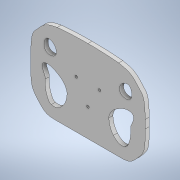
# Autodesk Inventor part: CF_base_3
Saved by Autodesk Inventor 2021 (Build 250183000, 183)
## iProperties
Created: 2020-12-19
Part Number: CF_base_3
Material: Generic
Document SubType Name: Modeling
Designer: capta
Density: 1 g/cm^3
Appearance: Default
Author: capta
Autodesk Inventor part; units mm, degrees
ref_plane "YZ Plane" through (0, 0, 0) normal (1, 0, 0) x (0, 1, 0)
ref_plane "XZ Plane" through (0, 0, 0) normal (0, 1, 0) x (-1, 0, 0)
ref_plane "XY Plane" through (0, 0, 0) normal (0, 0, 1) x (1, 0, 0)
sketch "Sketch1" plane through (0, 0, 0) normal (0, 0, 1) x (1, 0, 0)
  spline S0 degree 4 poles (-107.95, -1.5875) (-107.9501, -31.5854) (-105.1191, -42.7753) (-94.6432, -54.7155) (-85.2117, -65.4653) (-79.1753, -69.1153) (-72.5093, -71.2291) (-62.4463, -71.4375) knots 1 1 1 1 1 2 3 4 5 5 5 5 5
  line L0 (-62.4463, -71.4375) -> (62.4463, -71.4375)
  spline S1 degree 4 poles (62.4463, -71.4375) (72.5094, -71.2291) (79.1753, -69.1152) (85.2117, -65.4653) (94.6431, -54.7154) (105.119, -42.7752) (107.95, -31.5853) (107.95, -1.5875) knots 1 1 1 1 1 2 3 4 5 5 5 5 5
  spline S2 degree 4 poles (107.95, 14.2875) (107.3863, 39.342) (103.6451, 53.7014) (98.0708, 55.8562) (88.8552, 69.2477) (79.1753, 76.065) (71.1856, 78.9229) (57.9142, 81.444) knots 1 1 1 1 1 2 3 4 5 5 5 5 5
  spline S3 degree 2 poles (57.9142, 81.444) (34.5422, 83.9709) (0, 84.1375) knots 0 0 0 1 1 1
  spline S4 degree 2 poles (0, 84.1375) (-34.5422, 83.9709) (-57.9142, 81.444) knots 0 0 0 1 1 1
  spline S5 degree 4 poles (-57.9142, 81.444) (-71.1856, 78.9229) (-79.1753, 76.065) (-88.8553, 69.2477) (-98.0708, 55.8562) (-103.6451, 53.7014) (-107.3863, 39.342) (-107.95, 14.2875) knots 1 1 1 1 1 2 3 4 5 5 5 5 5
  circle A0 centre (21.971, 12.685) radius 2.3495
  circle A1 centre (0, -25.3699) radius 2.3495
  circle A2 centre (-21.971, 12.685) radius 2.3495
  spline S6 degree 3 poles (-80.6784, -14.2875) (-80.6812, -14.2577) (-80.6838, -14.2282) (-80.7753, -13.147) (-80.7131, -12.4053) (-80.7853, -10.6951) (-80.9388, -9.8114) (-81.7031, -7.8371) (-82.1979, -6.806) (-83.5598, -3.8976) (-84.4587, -1.9277) (-85.5995, 1.5041) (-85.8912, 2.9693) (-86.0776, 5.6047) (-86.0365, 6.8171) (-85.4697, 9.2744) (-84.856, 10.5052) (-82.0152, 12.1143) (-80.3762, 12.6519) (-76.1292, 13.0442) (-71.7337, 13.0635) (-64.2315, 10.4063) (-59.1205, 7.4272) knots 0.129586 0.129586 0.129586 0.129586 0.132442 0.132442 0.235411 0.235411 0.356197 0.356197 0.444476 0.444476 0.546294 0.546294 0.635178 0.635178 0.725825 0.725825 0.829514 0.829514 0.899662 0.899662 0.949831 1 1 1 1
  spline S7 degree 3 poles (-59.1205, 7.4272) (-54.9819, 5.1195) (-52.2606, 3.293) (-47.9423, -0.1336) (-46.4804, -1.6949) (-43.9371, -4.8912) (-42.926, -6.51) (-40.6921, -10.7647) (-39.8566, -13.2688) (-39.4632, -16.1749) (-39.4261, -16.8155) (-39.4429, -17.4332) knots 0 0 0 0 0.165028 0.165028 0.346804 0.346804 0.548512 0.548512 0.896468 0.896468 1 1 1 1
  spline S8 degree 3 poles (-39.4429, -17.4332) (-39.4826, -19.4908) (-39.7301, -32.3203) (-48.0538, -41.7892) knots 1 1 1 1 2 2 2 2
  spline S9 degree 4 poles (-79.4852, 52.6955) (-77.3336, 55.3925) (-74.2019, 55.3925) (-63.1401, 55.3925) (-56.2224, 36.3446) (-65.7167, 29.5906) (-74.478, 29.0411) (-84.5786, 32.7245) (-82.7866, 48.557) (-79.4852, 52.6955) knots 1 1 1 1 1 2 3 4 5 6 7 7 7 7 7
  spline S10 degree 4 poles (79.4852, 52.6955) (82.7866, 48.557) (84.5786, 32.7245) (74.478, 29.0411) (65.7167, 29.5906) (56.2224, 36.3446) (63.1401, 55.3925) (74.2019, 55.3925) (77.3336, 55.3925) (79.4852, 52.6955) knots 1 1 1 1 1 2 3 4 5 6 7 7 7 7 7
  line L1 (-107.95, -1.5875) -> (-107.95, 14.2875)
  line L2 (107.95, -1.5875) -> (107.95, 14.2875)
  line L3 (-68.9825, -49.9336) -> (-60.3634, -52.7472) construction
  line L4 (-60.3634, -52.7472) -> (-52.2222, -47.154) construction
  line L5 (-52.2222, -47.154) -> (-48.0538, -41.7892) construction
  spline S11 degree 3 poles (-68.9825, -49.9336) (-60.3634, -52.7472) (-52.2222, -47.154) (-48.0538, -41.7892) knots 1 1 1 1 2 2 2 2
  line L6 (-80.6784, -14.2875) -> (-80.7864, -23.0204) construction
  line L7 (-80.7864, -23.0204) -> (-80.1006, -35.5218) construction
  line L8 (-80.1006, -35.5218) -> (-75.8557, -41.1463) construction
  line L9 (-75.8557, -41.1463) -> (-74.2833, -48.2031) construction
  line L10 (-74.2833, -48.2031) -> (-68.9825, -49.9336) construction
  spline S12 degree 4 poles (-80.6784, -14.2875) (-80.7864, -23.0204) (-80.1006, -35.5218) (-75.8557, -41.1463) (-74.2833, -48.2031) (-68.9825, -49.9336) knots 1 1 1 1 1 2 3 3 3 3 3
  spline S13 degree 3 poles (39.4429, -17.4332) (39.4826, -19.4908) (39.7301, -32.3203) (48.0538, -41.7892) knots 1 1 1 1 2 2 2 2
  spline S14 degree 3 poles (80.6784, -14.2875) (80.6812, -14.2577) (80.6838, -14.2282) (80.7753, -13.147) (80.7131, -12.4053) (80.7853, -10.6951) (80.9388, -9.8114) (81.7031, -7.8371) (82.1979, -6.806) (83.5598, -3.8976) (84.4587, -1.9277) (85.5995, 1.5041) (85.8912, 2.9693) (86.0776, 5.6047) (86.0365, 6.8171) (85.4697, 9.2744) (84.856, 10.5052) (82.0152, 12.1143) (80.3762, 12.6519) (76.1292, 13.0442) (71.7337, 13.0635) (64.2315, 10.4063) (59.1205, 7.4272) knots 0.129586 0.129586 0.129586 0.129586 0.132442 0.132442 0.235411 0.235411 0.356197 0.356197 0.444476 0.444476 0.546294 0.546294 0.635178 0.635178 0.725825 0.725825 0.829514 0.829514 0.899662 0.899662 0.949831 1 1 1 1
  spline S15 degree 3 poles (59.1205, 7.4272) (54.9819, 5.1195) (52.2606, 3.293) (47.9423, -0.1336) (46.4804, -1.6949) (43.9371, -4.8912) (42.926, -6.51) (40.6921, -10.7647) (39.8566, -13.2688) (39.4632, -16.1749) (39.4261, -16.8155) (39.4429, -17.4332) knots 0 0 0 0 0.165028 0.165028 0.346804 0.346804 0.548512 0.548512 0.896468 0.896468 1 1 1 1
  line L11 (68.9825, -49.9336) -> (60.3634, -52.7472) construction
  line L12 (60.3634, -52.7472) -> (52.2222, -47.154) construction
  line L13 (52.2222, -47.154) -> (48.0538, -41.7892) construction
  spline S16 degree 3 poles (68.9825, -49.9336) (60.3634, -52.7472) (52.2222, -47.154) (48.0538, -41.7892) knots 1 1 1 1 2 2 2 2
  line L14 (80.6784, -14.2875) -> (80.7864, -23.0204) construction
  line L15 (80.7864, -23.0204) -> (80.1006, -35.5218) construction
  line L16 (80.1006, -35.5218) -> (75.8557, -41.1463) construction
  line L17 (75.8557, -41.1463) -> (74.2833, -48.2031) construction
  line L18 (74.2833, -48.2031) -> (68.9825, -49.9336) construction
  spline S17 degree 4 poles (80.6784, -14.2875) (80.7864, -23.0204) (80.1006, -35.5218) (75.8557, -41.1463) (74.2833, -48.2031) (68.9825, -49.9336) knots 1 1 1 1 1 2 3 3 3 3 3
  point P0 (-62.4463, -55.5625)
  point P1 (62.4463, -55.5625)
  constraints: 6 centre point, 6 end point, 1 parallel, 1 vertical, 64 other
extrude "Extrusion1" add sketch "Sketch1" along normal blind 7.62
sketch "Sketch2" plane through (0, 0, 7.62) normal (0, 0, 1) x (1, 0, 0)
  line L0 (0, 84.1375) -> (0, -71.4375)
  line L1 (-62.4463, -71.4375) -> (62.4463, -71.4375) projected
  line L2 (0, 6.35) -> (-27.4949, -8.5628)
  circle A0 centre (-21.971, 12.685) radius 2.3495 projected
  circle A1 centre (0, 6.35) radius 25.3746
  circle A2 centre (0, -19.0246) radius 2.3495
  circle A3 centre (21.975, 19.0373) radius 2.3495
  circle A4 centre (-21.975, 19.0373) radius 2.3495
  point P0 (0, 0)
  dimension "d4" = 50.7492
  dimension "d5" = 4.699
  dimension "d8" = 360
  constraints: 4 end point, 3 centre point, 2 midpoint, 1 coincident, 1 point on line, 1 vertical alignment, 9 other
  measures "d5" diameter of A2
extrude "Extrusion2" cut sketch "Sketch2" against normal blind 79.375 contours A3 A1 | A1 A3 | A4 A1 | A1 A4 | A2 A1 L0 | L0 A1 A2 | A1 A2 L0 | L0 A2 A1
sketch "Sketch3" plane through (0, 0, 7.62) normal (0, 0, 1) x (1, 0, 0)
  circle A0 centre (-21.971, 12.685) radius 2.3495
  circle A1 centre (21.971, 12.685) radius 2.3495
  circle A2 centre (0, -25.3699) radius 2.3495
  point P0 (0, 0)
  constraints: 3 centre point
extrude "Extrusion3" add sketch "Sketch3" against normal blind 7.62
body "Solid1"
